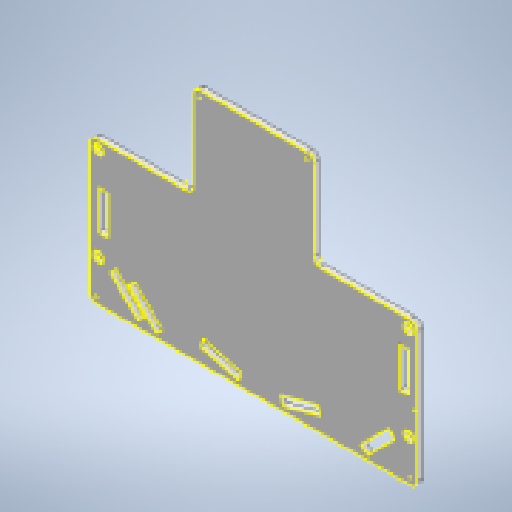
# Autodesk Inventor part: main_pcb
Saved by Autodesk Inventor 2023 (Build 270158000, 158)
## iProperties
Created: 2025-01-15
Part Number: main_pcb
Material: Ogólny
Document SubType Name: Modeling
Designer: kamil
Density: 1 g/cm^3
Appearance: Domyślna
Author: kamil
Autodesk Inventor part; units mm, degrees
ref_plane "YZ Plane" through (0, 0, 0) normal (1, 0, 0) x (0, 1, 0)
ref_plane "XZ Plane" through (0, 0, 0) normal (0, 1, 0) x (-1, 0, 0)
ref_plane "XY Plane" through (0, 0, 0) normal (0, 0, 1) x (1, 0, 0)
sketch "Szkic1" plane through (0, 0, 0) normal (0, 0, 1) x (1, 0, 0)
  circle A0 centre (-2, -7.4599) radius 1.4 projected
  circle A1 centre (-2, 20.4244) radius 1.4 projected
  circle A2 centre (-95, -7.4599) radius 1.4 projected
  circle A3 centre (-95, 20.4244) radius 1.4 projected
  line L0 (-98.5, 23.9244) -> (-98.5, -20.9244) projected
  line L1 (-97.6, 23.9244) -> (-97.6, -20.9244)
  line L2 (-98.5, -20.9244) -> (-91.5, -20.9244) projected
  line L3 (-98.5, 23.9244) -> (-91.5, 23.9244) projected
  line L4 (-98.5, -19.9244) -> (-91.5, -19.9244)
  line L5 (-91.5, -7.4599) -> (-91.5, -20.9244) projected
  line L6 (-97.6, 23.0244) -> (-92.3999, 23.0244)
  line L7 (-48.5, -51.6271) -> (-48.5, 68.0164)
  line L8 (-97.6, -19.9244) -> (-48.5, -19.9244)
  line L9 (-48.5, -19.9244) -> (-48.5, 23.0244)
  line L10 (-48.5, 23.0244) -> (-97.6, 23.0244)
  line L11 (-97.6, 23.0244) -> (-97.6, -19.9244)
  line L12 (0.6, -19.9244) -> (-48.5, -19.9244)
  line L13 (-48.5, 23.0244) -> (0.6, 23.0244)
  line L14 (0.6, 23.0244) -> (0.6, -19.9244)
  point P0 (0, 0)
  dimension "d0" = 0.9
  dimension "d1" = 1
  dimension "d2" = 0.9
  constraints: 22 end point, 5 point on line, 4 parallel, 2 horizontal, 2 symmetric about line, 1 perpendicular, 1 vertical, 2 other
  measures "d0" distance between parallel lines of L0 L1
  measures "d1" distance between parallel lines of L4 L2
  measures "d2" distance between parallel lines of L3 L6
extrude "Wyciągnięcie proste1" add sketch "Szkic1" along normal blind 1.6 contours L1 L6 L10 L7 L8 L4 | L7 L13 L14 L12
sketch "Szkic2" plane through (0, 0, 1.6) normal (0, 0, 1) x (1, 0, 0)
  line L0 (-29.5, 25.9244) -> (-29.5, 36.1286) projected
  line L1 (-31.5, 51.9244) -> (-65.5, 51.9244) projected
  line L2 (-67.5, 36.1286) -> (-67.5, 25.9244) projected
  line L3 (0.6, 23.0244) -> (-97.6, 23.0244) projected
  line L4 (-29.5, 23.0244) -> (-67.5, 23.0244)
  line L5 (-67.5, 23.0244) -> (-67.5, 51.9244)
  line L6 (-67.5, 51.9244) -> (-29.5, 51.9244)
  line L7 (-29.5, 51.9244) -> (-29.5, 23.0244)
  line L8 (-30.4, 23.9244) -> (-66.6, 23.9244)
  line L9 (-66.6, 23.9244) -> (-66.6, 51.0244)
  line L10 (-66.6, 51.0244) -> (-30.4, 51.0244)
  line L11 (-30.4, 51.0244) -> (-30.4, 23.9244)
  line L12 (-30.4, 23.9244) -> (-30.4, 23.0244)
  line L13 (-66.6, 23.9244) -> (-66.6, 23.0244)
  point P0 (0, 0)
  point P1 (-67.5, 37.4744)
  point P2 (-29.5, 37.4744)
  point P3 (-29.5, 31.0265)
  point P4 (-48.5, 51.9244)
  dimension "d5" = 0.9
  constraints: 20 end point, 4 midpoint, 4 parallel, 4 perpendicular, 3 point on line, 2 vertical alignment, 1 horizontal, 1 horizontal alignment, 3 other
  measures "d5" distance between parallel lines of L7 L11
extrude "Wyciągnięcie proste2" add sketch "Szkic2" against normal blind 1.6 contours L3 L13 L8 L12 | L8 L9 L10 L11
sketch "Szkic3" plane through (0, 0, 1.6) normal (0, 0, 1) x (1, 0, 0)
  line L0 (-94.4, -0.5756) -> (-94.4, 10.1244) projected
  line L1 (-94.4, 10.1244) -> (-92.8, 10.1244) projected
  line L2 (-92.8, 10.1244) -> (-92.8, -0.5756) projected
  line L3 (-94.4, -0.5756) -> (-92.8, -0.5756) projected
  line L4 (-77.7433, -17.9244) -> (-76.6119, -16.7931) projected
  line L5 (-77.7433, -17.9244) -> (-85.3094, -10.3584) projected
  line L6 (-84.178, -9.227) -> (-76.6119, -16.7931) projected
  line L7 (-85.3094, -10.3584) -> (-84.178, -9.227) projected
  line L8 (-63.3019, -13.6096) -> (-52.9665, -16.379) projected
  line L9 (-63.716, -15.1551) -> (-63.3019, -13.6096) projected
  line L10 (-53.3806, -17.9244) -> (-63.716, -15.1551) projected
  line L11 (-29.1305, -15.1551) -> (-39.4659, -17.9244) projected
  line L12 (-39.88, -16.379) -> (-29.5446, -13.6096) projected
  line L13 (-29.1305, -15.1551) -> (-29.5446, -13.6096) projected
  line L14 (-39.4659, -17.9244) -> (-39.88, -16.379) projected
  line L15 (-53.3806, -17.9244) -> (-52.9665, -16.379) projected
  line L16 (-14.4607, -17.9244) -> (-15.592, -16.7931) projected
  line L17 (-15.592, -16.7931) -> (-8.026, -9.227) projected
  line L18 (-6.8946, -10.3584) -> (-14.4607, -17.9244) projected
  line L19 (-6.8946, -10.3584) -> (-8.026, -9.227) projected
  line L20 (-2.6, 14.4244) -> (-4.2, 14.4244) projected
  line L21 (-4.2, 3.7244) -> (-4.2, 14.4244) projected
  line L22 (-2.6, 3.7244) -> (-4.2, 3.7244) projected
  line L23 (-2.6, 14.4244) -> (-2.6, 3.7244) projected
  line L24 (-92.3, -1.0756) -> (-92.3, 10.6244)
  line L25 (-92.3, 10.6244) -> (-94.9, 10.6244)
  line L26 (-94.9, 10.6244) -> (-94.9, -1.0756)
  line L27 (-94.9, -1.0756) -> (-92.3, -1.0756)
  line L28 (-75.9048, -16.7931) -> (-77.7433, -18.6316)
  line L29 (-77.7433, -18.6316) -> (-86.0165, -10.3584)
  line L30 (-86.0165, -10.3584) -> (-84.178, -8.5199)
  line L31 (-84.178, -8.5199) -> (-75.9048, -16.7931)
  line L32 (-52.3541, -16.0254) -> (-63.6554, -12.9972)
  line L33 (-63.6554, -12.9972) -> (-64.3284, -15.5086)
  line L34 (-64.3284, -15.5086) -> (-53.027, -18.5368)
  line L35 (-53.027, -18.5368) -> (-52.3541, -16.0254)
  line L36 (-29.1911, -12.9972) -> (-40.4924, -16.0254)
  line L37 (-40.4924, -16.0254) -> (-39.8195, -18.5368)
  line L38 (-39.8195, -18.5368) -> (-28.5181, -15.5086)
  line L39 (-28.5181, -15.5086) -> (-29.1911, -12.9972)
  line L40 (-8.026, -8.5199) -> (-16.2991, -16.7931)
  line L41 (-16.2991, -16.7931) -> (-14.4607, -18.6316)
  line L42 (-14.4607, -18.6316) -> (-6.1875, -10.3584)
  line L43 (-6.1875, -10.3584) -> (-8.026, -8.5199)
  line L44 (-4.7, 3.2244) -> (-4.7, 14.9244)
  line L45 (-4.7, 14.9244) -> (-2.1, 14.9244)
  line L46 (-2.1, 14.9244) -> (-2.1, 3.2244)
  line L47 (-2.1, 3.2244) -> (-4.7, 3.2244)
  point P0 (0, 0)
  dimension "d8" = 0.5
  dimension "d9" = 0.5
  dimension "d10" = 0.5
  dimension "d11" = 0.5
  dimension "d12" = 0.5
  dimension "d13" = 0.5
  constraints: 48 end point, 18 other
  measures "d8" distance between parallel lines of L2 L24
  measures "d9" distance between parallel lines of L6 L31
  measures "d10" distance between parallel lines of L8 L32
  measures "d11" distance between parallel lines of L12 L36
  measures "d12" distance between parallel lines of L17 L40
  measures "d13" distance between parallel lines of L22 L47
extrude "Wyciągnięcie proste3" cut sketch "Szkic3" against normal blind 1.6 contours L0 L1 L2 L3 | L5 L7 L6 L4 | L8 L15 L10 L9 | L11 L14 L12 L13 | L16 L17 L19 L18 | L23 L22 L21 L20 | L27 L26 L25 L24 | L28 L29 L30 L31 | L35 L34 L33 L32 | L39 L38 L37 L36 | L43 L42 L41 L40 | L44 L45 L46 L47
fillet "Zaokrąglenie1" radius 2 8 edges at (-66.6, 51.0244, 0.8) (-66.6, 23.0244, 0.8) (-97.6, 23.0244, 0.8) (-97.6, -19.9244, 0.8) (0.6, 23.0244, 0.8) (0.6, -19.9244, 0.8) (-30.4, 23.0244, 0.8) (-30.4, 51.0244, 0.8)
sketch "Szkic4" plane through (0, 0, 1.6) normal (0, 0, 1) x (1, 0, 0)
  circle A0 centre (-2, 20.4244) radius 1.4 projected
  circle A1 centre (-2, -7.4599) radius 1.4 projected
  circle A2 centre (-95, 20.4244) radius 1.4 projected
  circle A3 centre (-95, -7.4599) radius 1.4 projected
  point P0 (0, 0)
hole "Otwór1" at (-2, 20.4244, 1.6) at (-2, -7.4599, 1.6) at (-95, 20.4244, 1.6) at (-95, -7.4599, 1.6) direction (0, 0, -1) diameter 3 end through all
sketch "Szkic5" plane through (0, 0, 1.6) normal (0, 0, 1) x (1, 0, 0)
  circle A0 centre (-95, 20.4244) radius 1.5 projected
  circle A1 centre (-2, 20.4244) radius 1.5 projected
  circle A2 centre (-2, -7.4599) radius 1.5 projected
  circle A3 centre (-95, -7.4599) radius 1.5 projected
  arc A4 (-30.4, 49.0244) -> (-32.4, 51.0244) centre (-32.4, 49.0244) ccw projected
  line L0 (-32.4, 51.0244) -> (-64.6, 51.0244) projected
  arc A5 (-64.6, 51.0244) -> (-66.6, 49.0244) centre (-64.6, 49.0244) ccw projected
  line L1 (-66.6, 49.0244) -> (-66.6, 25.0244) projected
  arc A6 (-68.6, 23.0244) -> (-66.6, 25.0244) centre (-68.6, 25.0244) ccw projected
  line L2 (-68.6, 23.0244) -> (-95.6, 23.0244) projected
  arc A7 (-95.6, 23.0244) -> (-97.6, 21.0244) centre (-95.6, 21.0244) ccw projected
  line L3 (-97.6, 21.0244) -> (-97.6, -17.9244) projected
  arc A8 (-97.6, -17.9244) -> (-95.6, -19.9244) centre (-95.6, -17.9244) ccw projected
  line L4 (-95.6, -19.9244) -> (-1.4, -19.9244) projected
  arc A9 (-1.4, -19.9244) -> (0.6, -17.9244) centre (-1.4, -17.9244) ccw projected
  line L5 (0.6, -17.9244) -> (0.6, 21.0244) projected
  arc A10 (0.6, 21.0244) -> (-1.4, 23.0244) centre (-1.4, 21.0244) ccw projected
  line L6 (-1.4, 23.0244) -> (-28.4, 23.0244) projected
  arc A11 (-30.4, 25.0244) -> (-28.4, 23.0244) centre (-28.4, 25.0244) ccw projected
  line L7 (-30.4, 25.0244) -> (-30.4, 49.0244) projected
  line L8 (-94.9, -1.0756) -> (-94.9, 10.6244) projected
  line L9 (-94.9, 10.6244) -> (-92.3, 10.6244) projected
  line L10 (-92.3, 10.6244) -> (-92.3, -1.0756) projected
  line L11 (-92.3, -1.0756) -> (-94.9, -1.0756) projected
  line L12 (-6.1875, -10.3584) -> (-14.4607, -18.6316) projected
  line L13 (-14.4607, -18.6316) -> (-16.2991, -16.7931) projected
  line L14 (-16.2991, -16.7931) -> (-8.026, -8.5199) projected
  line L15 (-8.026, -8.5199) -> (-6.1875, -10.3584) projected
  line L16 (-28.5181, -15.5086) -> (-39.8195, -18.5368) projected
  line L17 (-39.8195, -18.5368) -> (-40.4924, -16.0254) projected
  line L18 (-40.4924, -16.0254) -> (-29.1911, -12.9972) projected
  line L19 (-29.1911, -12.9972) -> (-28.5181, -15.5086) projected
  line L20 (-77.7433, -18.6316) -> (-86.0165, -10.3584) projected
  line L21 (-86.0165, -10.3584) -> (-84.178, -8.5199) projected
  line L22 (-84.178, -8.5199) -> (-75.9048, -16.7931) projected
  line L23 (-75.9048, -16.7931) -> (-77.7433, -18.6316) projected
  line L24 (-4.7, 14.9244) -> (-2.1, 14.9244) projected
  line L25 (-2.1, 14.9244) -> (-2.1, 3.2244) projected
  line L26 (-2.1, 3.2244) -> (-4.7, 3.2244) projected
  line L27 (-4.7, 3.2244) -> (-4.7, 14.9244) projected
  line L28 (-53.027, -18.5368) -> (-64.3284, -15.5086) projected
  line L29 (-64.3284, -15.5086) -> (-63.6554, -12.9972) projected
  line L30 (-63.6554, -12.9972) -> (-52.3541, -16.0254) projected
  line L31 (-52.3541, -16.0254) -> (-53.027, -18.5368) projected
  line L32 (-91.5, -9.7839) -> (-83.2269, -18.057)
  line L33 (-83.2269, -18.057) -> (-81.3884, -16.2185)
  line L34 (-81.3884, -16.2185) -> (-89.6615, -7.9454)
  line L35 (-89.6615, -7.9454) -> (-91.5, -9.7839)
  line L36 (-91.5, -7.4599) -> (-91.5, -20.9244) projected
  line L37 (-77.7433, -18.057) -> (-77.7433, -19.9244) construction
  line L38 (-83.2269, -18.057) -> (-83.2269, -19.9244) construction
  point P0 (0, 0)
  constraints: 12 end point, 4 parallel, 4 perpendicular, 3 point on line, 1 vertical
extrude "Wyciągnięcie proste4" cut sketch "Szkic5" against normal through all contours L35 L34 L33 L32
